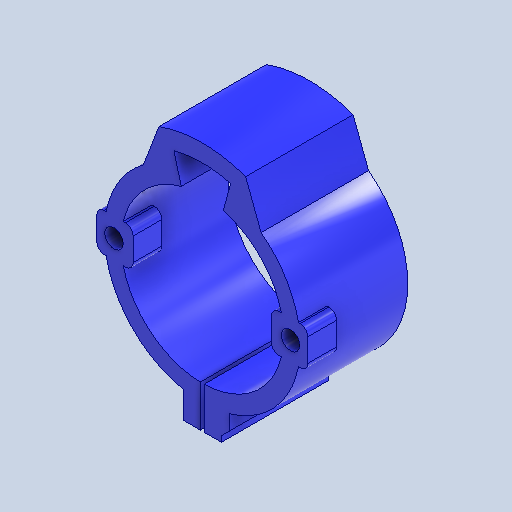
# Autodesk Inventor part: 軸止め
Saved by Autodesk Inventor 2022 (Build 260153000, 153)
## iProperties
Created: 2019-12-20
Part Number: 軸止め
Material: ABS プラスチック
Document SubType Name: Modeling
Designer: Hagihara Yuya
Density: 0.673187 g/cm^3
Appearance: 青 - 壁塗料 - 光沢
Mass: 15.58 g
Surface Area: 121.799 cm^2
Volume: 23.1436 cm^3
Author: Hagihara Yuya
Autodesk Inventor part; units mm, degrees
ref_plane "YZ Plane" through (0, 0, 0) normal (1, 0, 0) x (0, 1, 0)
ref_plane "XZ Plane" through (0, 0, 0) normal (0, 1, 0) x (-1, 0, 0)
ref_plane "XY Plane" through (0, 0, 0) normal (0, 0, 1) x (1, 0, 0)
sketch "スケッチ1" plane through (0, 0, 0) normal (0, 0, 1) x (1, 0, 0)
  line L0 (0, 0) -> (10, 0)
  line L1 (10, 0) -> (10, 32.05)
  line L2 (10, 32.05) -> (0, 32.05)
  line L3 (0, 32.05) -> (0, 0)
  circle A0 centre (5, 32.05) radius 25.55
  arc A1 (16.3038, 63.1068) -> (-6.3038, 63.1068) centre (5, 32.05) ccw
  line L4 (5, 32.05) -> (16.3038, 63.1068) construction
  line L5 (5, 32.05) -> (-6.3038, 63.1068) construction
  line L6 (-6.3038, 63.1068) -> (-3.7386, 56.0591)
  line L7 (16.3038, 63.1068) -> (13.7386, 56.0591)
  arc A2 (12.3893, 59.6272) -> (-2.3893, 59.6272) centre (5, 32.05) ccw
  arc A3 (10.4481, 52.3827) -> (-0.4481, 52.3827) centre (5, 32.05) ccw
  line L8 (-2.3893, 59.6272) -> (-0.4481, 52.3827)
  line L9 (12.3893, 59.6272) -> (10.4481, 52.3827)
  point P0 (0, 6.994)
  point P1 (10, 6.994)
  point P2 (5, 65.1)
  point P3 (5, 60.6)
  dimension "d0" = 32.05
  dimension "d1" = 51.1
  dimension "d27" = 10
  dimension "d28" = 5
  dimension "d43" = 21.05
  dimension "d44" = 7.5
  dimension "d45" = 4.5
  dimension "d46" = 30
  dimension "d47" = 5
  constraints: 20 end point, 10 point on circle, 4 centre point, 3 coincident, 2 line through centre, 2 midpoint, 2 parallel, 2 point on line, 2 vertical alignment, 1 horizontal, 1 perpendicular
  measures "d0" distance of L2.end L0.start
  measures "d1" diameter of A0
  measures "d27" distance of L1.end L2.end
  measures "d28" distance of A0.centre L2.end
  measures "d43" radius of A3
  measures "d44" distance of L9.start L9.end
  measures "d45" radial gap between concentric circles of A1 A2
  measures "d46" angle of L9 L8
  measures "d47" angle of L9 L4
extrude "押し出し1" add sketch "スケッチ1" along normal blind 28 contours L3 A0 L1 L0 | A0 L8 A3 L9 L1 L2 L3 | L3 L2 L1 A0 | L6 A1 L7 A0 L9 A2 L8
sketch "スケッチ2" plane through (0, 0, 28) normal (0, 0, 1) x (1, 0, 0)
  arc A0 (10, 6.994) -> (0, 6.994) centre (5, 32.05) ccw projected
  point P0 (0, 0)
  constraints: 1 coincident
hole "穴1" at (5, 32.05, 28) direction (0, 0, -1) diameter 42.4 end through all
sketch "スケッチ3" plane through (0, 0, 28) normal (0, 0, 1) x (1, 0, 0)
  line L0 (0, 0) -> (10, 0) projected
  line L1 (4.5, 0) -> (5.5, 0)
  line L2 (5.5, 0) -> (5.5, 32.05)
  line L3 (5.5, 32.05) -> (4.5, 32.05)
  line L4 (4.5, 32.05) -> (4.5, 0)
  line L5 (0, 6.994) -> (0, 0) projected
  arc A0 (-0.487, 52.5276) -> (10.487, 52.5276) centre (5, 32.05) ccw projected
  point P0 (5, 0)
  point P1 (5, 0)
  dimension "d14" = 1
  constraints: 8 end point, 3 midpoint, 2 coincident, 2 parallel, 1 horizontal, 1 perpendicular, 1 point on line
  measures "d14" distance of L2.end L3.end
extrude "押し出し2" cut sketch "スケッチ3" against normal up to surface (28 mm away)
sketch "スケッチ4" plane through (10, 0, 0) normal (1, 0, 0) x (0, 0, -1)
  circle A0 centre (-14, 4) radius 1.5
  line L0 (0, 0) -> (-28, 0) projected
  line L1 (0, 0) -> (0, 6.994) projected
  line L2 (-14, 0) -> (-14, 10)
  point P0 (0, 10)
  dimension "d17" = 4
  dimension "d19" = 3
  constraints: 2 end point, 1 centre point, 1 midpoint, 1 point on line, 1 vertical
  measures "d17" distance from line of L0 A0.centre
  measures "d19" diameter of A0
hole "穴2" at (10, 4, 14) direction (-1, 0, 0) diameter 4.4 end through all
sketch "スケッチ7" plane through (10, 0, 0) normal (1, 0, 0) x (0, 0, -1)
  circle A0 centre (-14, 4) radius 2.2 projected
  line L0 (-14, 8.1569) -> (-10.4, 6.0785)
  line L1 (-10.4, 6.0785) -> (-10.4, 1.9215)
  line L2 (-10.4, 1.9215) -> (-14, -0.1569)
  line L3 (-14, -0.1569) -> (-17.6, 1.9215)
  line L4 (-17.6, 1.9215) -> (-17.6, 6.0785)
  line L5 (-17.6, 6.0785) -> (-14, 8.1569)
  line L6 (-28, 10.8559) -> (-28, 0) projected
  line L7 (0, 0) -> (0, 6.994) projected
  line L8 (-28, 10.8559) -> (0, 10.8559)
  line L9 (0, 10.8559) -> (0, 3.497)
  line L10 (0, 3.497) -> (-28, 3.497)
  line L11 (-28, 3.497) -> (-28, 10.8559)
  point P0 (-10.4, 3.497)
  point P1 (-28, 3.497)
  point P2 (-17.6, 3.497)
  dimension "d35" = 7.2
  constraints: 20 end point, 2 parallel, 1 coincident, 1 horizontal, 1 horizontal alignment, 1 midpoint, 1 perpendicular, 13 other
  measures "d35" distance between parallel lines of L0 L3
extrude "押し出し5" add sketch "スケッチ7" along normal blind 2 contours L10 L6 L8 L9 L7 L1 L0 L5 L4
chamfer "面取り1" distance 2 angle 45 2 edges at (10, 3.497, 22.8) (10, 3.497, 5.2)
chamfer "面取り2" distance 7.5 angle 45 2 edges at (-3.7386, 56.0591, 14) (13.7386, 56.0591, 14)
sketch "スケッチ8" plane through (0, 0, 28) normal (0, 0, 1) x (1, 0, 0)
  arc A0 (12, 7.4776) -> (20.3335, 52.4874) centre (5, 32.05) ccw projected
  line L0 (30.056, 37.05) -> (32.5, 37.05)
  line L1 (32.5, 37.05) -> (32.5, 27.05)
  line L2 (32.5, 27.05) -> (30.056, 27.05)
  line L3 (30.056, 27.05) -> (30.056, 37.05)
  arc A1 (-10.3335, 52.4874) -> (0, 6.994) centre (5, 32.05) ccw projected
  line L4 (-20.056, 37.05) -> (-22.5, 37.05)
  line L5 (-22.5, 37.05) -> (-22.5, 27.05)
  line L6 (-22.5, 27.05) -> (-20.056, 27.05)
  line L7 (-20.056, 27.05) -> (-20.056, 37.05)
  arc A2 (-10.3335, 52.4874) -> (0, 6.994) centre (5, 32.05) ccw projected
  line L8 (30.056, 37.05) -> (23.0125, 37.05)
  line L9 (23.0125, 37.05) -> (23.0125, 27.05)
  line L10 (23.0125, 27.05) -> (30.056, 27.05)
  line L11 (30.056, 27.05) -> (30.056, 37.05)
  line L12 (-20.056, 37.05) -> (-13.0125, 37.05)
  line L13 (-13.0125, 37.05) -> (-13.0125, 27.05)
  line L14 (-13.0125, 27.05) -> (-20.056, 27.05)
  line L15 (-20.056, 27.05) -> (-20.056, 37.05)
  arc A3 (12, 7.4776) -> (20.3335, 52.4874) centre (5, 32.05) ccw projected
  point P0 (0, 0)
  dimension "d51" = 55
  dimension "d52" = 10
  dimension "d57" = 36.025
  constraints: 32 end point, 8 parallel, 4 horizontal, 4 perpendicular, 4 point on circle, 3 point on line, 2 collinear
  measures "d51" distance between parallel lines of L1 L5
  measures "d52" distance of L0.end L1.end
  measures "d57" distance between parallel lines of L13 L9
extrude "押し出し6" add sketch "スケッチ8" against normal blind 7.5
sketch "スケッチ9" plane through (0, 0, 28) normal (0, 0, 1) x (1, 0, 0)
  line L0 (32.5, 27.05) -> (32.5, 37.05) projected
  arc A0 (5.5, 10.8559) -> (10.487, 52.5276) centre (5, 32.05) ccw projected
  point P0 (0, 0)
  point P1 (-18.0125, 32.05)
  point P2 (28.0125, 32.05)
  point P3 (32.5, 32.05)
  dimension "d55" = 46.025
  dimension "d56" = 23.0125
  constraints: 2 horizontal alignment, 1 midpoint
  measures "d55" distance of point (-18.013, 32.05) point (28.012, 32.05)
  measures "d56" distance of point (28.012, 32.05) A0.centre
hole "穴3" at (-18.0125, 32.05, 28) at (28.0125, 32.05, 28) direction (0, 0, -1) diameter 4.8 depth 5
fillet "フィレット1" radius 2 8 edges at (-22.5, 37.05, 24.25) (-22.5, 27.05, 24.25) (-13.0125, 37.05, 24.25) (-13.0125, 27.05, 24.25) (32.5, 37.05, 24.25) (32.5, 27.05, 24.25) (23.0125, 37.05, 24.25) (23.0125, 27.05, 24.25)
equation "\"d28\" = 0.5 * d27"
equation "\"d56\" = 0.5 * d55"
